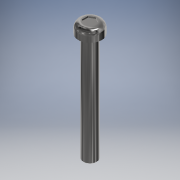
# Autodesk Inventor part: bolt m5
Saved by Autodesk Inventor 2018 (Build 220112000, 112)
## iProperties
Created: 2023-12-05
Part Number: bolt m5
Material: Generic
Document SubType Name: Modeling
Designer: DDUGKY
Density: 1 g/cm^3
Appearance: Steel - Polished
Author: DDUGKY
Autodesk Inventor part; units mm, degrees
ref_plane "YZ Plane" through (0, 0, 0) normal (1, 0, 0) x (0, 1, 0)
ref_plane "XZ Plane" through (0, 0, 0) normal (0, 1, 0) x (-1, 0, 0)
ref_plane "XY Plane" through (0, 0, 0) normal (0, 0, 1) x (1, 0, 0)
sketch "Sketch1" plane through (0, 0, 0) normal (0, 0, 1) x (1, 0, 0)
  circle A0 centre (0, 0) radius 2.5
  dimension "d0" = 5
  constraints: 1 centre point, 1 coincident
  measures "d0" diameter of A0
extrude "Extrusion1" add sketch "Sketch1" against normal blind 40
sketch "Sketch2" plane through (0, 0, 0) normal (0, 0, 1) x (1, 0, 0)
  circle A0 centre (0, 0) radius 4.3
  dimension "d3" = 8.6
  constraints: 1 centre point, 1 coincident
  measures "d3" diameter of A0
extrude "Extrusion2" add sketch "Sketch2" along normal blind 4
fillet "Fillet1" radius 2 1 edges at (-4.3, 0, 4)
sketch "Sketch3" plane through (0, 0, 4) normal (0, 0, 1) x (1, 0, 0)
  line L0 (0, -2.162) -> (-1.8723, -1.081)
  line L1 (-1.8723, -1.081) -> (-1.8723, 1.081)
  line L2 (-1.8723, 1.081) -> (0, 2.162)
  line L3 (0, 2.162) -> (1.8723, 1.081)
  line L4 (1.8723, 1.081) -> (1.8723, -1.081)
  line L5 (1.8723, -1.081) -> (0, -2.162)
  point P0 (0, 0)
  point P1 (0, 0)
  constraints: 12 end point, 1 coincident, 13 other
extrude "Extrusion3" cut sketch "Sketch3" against normal blind 0.5
chamfer "Chamfer1" distance 0.5 angle 45 1 edges at (-2.5, 0, -40)
body "Solid1"
